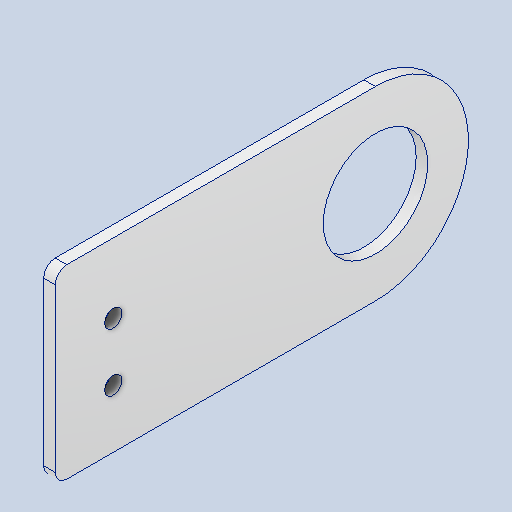
# Autodesk Inventor part: dribl-v1-Plate-4
Saved by Autodesk Inventor 2025.2 (Build 292293000, 293)
## iProperties
Created: 2025-01-07
Part Number: dribl-v1-Plate-4
Material: アルミニウム 6061
Document SubType Name: Modeling
Designer: haruy
Density: 2.7 g/cm^3
Appearance: アルミニウム - フラット
Mass: 10.2561 g
Surface Area: 43.346 cm^2
Volume: 3.79856 cm^3
Author: haruy
Autodesk Inventor part; units mm, degrees
ref_plane "YZ Plane" through (0, 0, 0) normal (1, 0, 0) x (0, 1, 0)
ref_plane "XZ Plane" through (0, 0, 0) normal (0, 1, 0) x (-1, 0, 0)
ref_plane "XY Plane" through (0, 0, 0) normal (0, 0, 1) x (1, 0, 0)
derived "dribl-v1-ASP-Base.ipt"
sketch "スケッチ3" plane through (420, -432.3334, -303) normal (1, 0, 0) x (0, 0, -1)
  line L0 (20, 0) -> (20, 1308) projected
  line L1 (20, 102) -> (425, 102) projected
  line L2 (425, 102) -> (425, 122) projected
  line L3 (425, 122) -> (20, 122) projected
  line L4 (20, 122) -> (20, 102) projected
  circle A0 centre (55.18, 149) radius 21 projected
  circle A1 centre (55.18, 191) radius 16 projected
  circle A2 centre (55.18, 191) radius 13.68 projected
  line L5 (0, 0) -> (20, 0) projected
  line L6 (0, 0) -> (20, 0) projected
  line L7 (0, 0) -> (484, 0) projected
  line L8 (484, 0) -> (484, -20) projected
  line L9 (484, -20) -> (0, -20) projected
  line L10 (0, -20) -> (0, 0) projected
  line L11 (75.18, 1308) -> (94.3557, 1313.6826) projected
  line L12 (94.3557, 1313.6826) -> (480.203, 11.6512) projected
  line L13 (480.203, 11.6512) -> (461.0273, 5.9686) projected
  line L14 (461.0273, 5.9686) -> (75.18, 1308) projected
  line L15 (0, 1308) -> (0, 0) projected
  line L16 (0, 207) -> (55.18, 207) projected
  line L17 (76.18, 149) -> (76.18, 102) projected
  line L18 (76.18, 149) -> (76.18, 207) projected
  line L19 (76.18, 207) -> (55.18, 207) projected
  circle A3 centre (10, 195) radius 1.5 projected
  circle A4 centre (10, 185) radius 1.5 projected
  line L20 (55.18, 175) -> (0, 175) projected
  circle A5 centre (30, 112) radius 1.5 projected
  circle A6 centre (50, 112) radius 1.5 projected
  line L21 (20, 102) -> (0, 102) projected
  circle A7 centre (10, 112) radius 1.5 projected
  circle A8 centre (10, 132) radius 1.5 projected
  circle A9 centre (55.18, 1292) radius 16 projected
  line L22 (20, 1308) -> (0, 1308) projected
  line L23 (0, 1308) -> (55.18, 1308) projected
  line L24 (55.18, 1276) -> (0, 1276) projected
  line L25 (55.18, 1308) -> (75.18, 1308) projected
  circle A10 centre (55.18, 191) radius 9
  circle A11 centre (55.18, 1292) radius 7.5 projected
  line L26 (55.18, 1276) -> (84.663, 1276) projected
  circle A12 centre (10, 1296) radius 1.5 projected
  circle A13 centre (10, 1286) radius 1.5 projected
  circle A14 centre (87.6092, 1301.2534) radius 1.5 projected
  circle A15 centre (90.4504, 1291.6656) radius 1.5 projected
  line L27 (84.663, 1276) -> (103.8387, 1281.6826) projected
  line L28 (20, 40) -> (40, 0) projected
  line L29 (40, 0) -> (40, -20) projected
  line L30 (20, 40) -> (0, 40) projected
  circle A16 centre (10, 10) radius 1.5 projected
  circle A17 centre (10, 20) radius 1.5 projected
  circle A18 centre (10, 30) radius 1.5 projected
  circle A19 centre (10, -10) radius 1.5 projected
  circle A20 centre (20, -10) radius 1.5 projected
  circle A21 centre (30, -10) radius 1.5 projected
  line L31 (0, 0) -> (0, 40) projected
  line L32 (454, 0) -> (454, -20) projected
  line L33 (452.5035, 34.7322) -> (471.6792, 40.4147) projected
  line L34 (461.0273, 5.9686) -> (462.7961, 0) projected
  line L35 (480.203, 11.6512) -> (484, 0) projected
  circle A22 centre (464, -10) radius 1.5 projected
  circle A23 centre (474, -10) radius 1.5 projected
  circle A24 centre (467.7739, 18.3977) radius 1.5 projected
  circle A25 centre (464.9326, 27.9856) radius 1.5 projected
  circle A26 centre (405, 112) radius 1.5 projected
  circle A27 centre (415, 112) radius 1.5 projected
  line L36 (425, 122) -> (426.6423, 122) projected
  line L37 (425, 102) -> (432.5691, 102) projected
  line L38 (426.6423, 122) -> (447.502, 122) projected
  circle A28 centre (439.9292, 112.3588) radius 1.5 projected
  circle A29 centre (442.7705, 102.7709) radius 1.5 projected
  line L39 (436.024, 90.3417) -> (455.1997, 96.0243) projected
  line L40 (395, 122) -> (395, 102) projected
  point P0 (-303, 432.3334)
  point P1 (470.6152, 8.8099)
  dimension "d1" = 18
  constraints: 1 centre point, 1 coincident, 1 horizontal alignment
  measures "d1" diameter of A10
extrude "押し出し1" add sketch "スケッチ3" against normal blind 2 contours L20 L15 L16 L0 | L0 L16 A1 L20 | A1 | A2
fillet "フィレット1" radius 2 2 edges at (419, -225.3334, -303) (419, -257.3334, -303)
